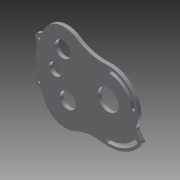
# Autodesk Inventor part: front plate
Saved by Autodesk Inventor 2012 (Build 160160000, 160)
## iProperties
Created: 2012-02-07
Part Number: front plate
Material: Default
Document SubType Name: Modeling
Designer: Antonella Wilby
Density: 1 g/cm^3
Author: Antonella Wilby
Autodesk Inventor part; units mm, degrees
ref_plane "YZ Plane" through (0, 0, 0) normal (1, 0, 0) x (0, 1, 0)
ref_plane "XZ Plane" through (0, 0, 0) normal (0, 1, 0) x (-1, 0, 0)
ref_plane "XY Plane" through (0, 0, 0) normal (0, 0, 1) x (1, 0, 0)
sketch "Sketch1" plane through (0, 0, 0) normal (0, 0, 1) x (1, 0, 0)
  line L0 (-198.2999, 0) -> (115.1427, 0) projected
  line L1 (0, -203.8942) -> (0, 193.807) projected
  circle A0 centre (0, 0) radius 53.975 construction
  circle A1 centre (0, 0) radius 19.05
  arc A2 (50.8401, -18.1268) -> (-4.087, 53.82) centre (0, 0) ccw
  line L2 (51.6197, -23.9016) -> (59.4633, -35.1034)
  arc A3 (50.8401, -18.1268) -> (51.6197, -23.9016) centre (56.8213, -20.2594) ccw
  line L3 (0, 0) -> (-57.7807, -26.9436) construction
  circle A4 centre (0, 0) radius 53.975 construction
  circle A5 centre (-95.7467, 0) radius 11.1125
  circle A6 centre (-73.1257, -37.5239) radius 14.2875
  circle A7 centre (-82.0671, 38.2685) radius 14.2875
  arc A8 (-56.7688, 67.6544) -> (-118.11, 48.895) centre (-79.7827, 33.238) ccw
  arc A9 (-118.11, -50.8) -> (-59.2151, -78.8871) centre (-77.6901, -41.8358) ccw
  arc A10 (-12.3378, -71.9752) -> (-59.2151, -78.8871) centre (-25.2121, -147.0797) ccw
  circle A11 centre (0, 0) radius 16.51 construction
  line L4 (0, 0) -> (-82.0671, 38.2685) construction
  circle A12 centre (-125.73, 34.29) radius 6.35 construction
  circle A13 centre (-125.73, -34.29) radius 6.35 construction
  line L5 (0, 0) -> (-34.422, 64.7383) construction
  line L6 (0, 0) -> (-56.7688, 67.6544) construction
  arc A14 (-127.2193, 41.2768) -> (-132.0785, 31.0144) centre (-125.73, 34.29) ccw
  arc A15 (-130.3268, 13.3001) -> (-130.3268, -13.3001) centre (-83.9357, 0) ccw
  arc A16 (-130.3268, 13.3001) -> (-132.0785, 31.0144) centre (-153.5223, 19.9501) ccw
  arc A17 (-132.0785, -31.0144) -> (-127.4503, -41.2235) centre (-125.73, -34.29) ccw
  arc A18 (-132.0785, -31.0144) -> (-130.3268, -13.3001) centre (-153.5223, -19.9501) ccw
  arc A19 (-118.11, -50.8) -> (-127.4503, -41.2235) centre (-130.5087, -53.5498) ccw
  arc A20 (-127.2193, 41.2768) -> (-118.11, 48.895) centre (-129.8669, 53.6978) ccw
  line L7 (-198.2999, 0) -> (115.1427, 0) projected
  line L8 (0, 193.807) -> (0, -203.8942) projected
  line L9 (-118.11, -50.8) -> (0, -50.8) construction
  arc A21 (-12.3378, -71.9752) -> (59.4295, -42.4357) centre (0, 0) ccw
  arc A22 (59.4295, -42.4357) -> (59.4633, -35.1034) centre (54.2617, -38.7456) ccw
  line L10 (0, 0) -> (41.8854, -59.8186) construction
  line L11 (-118.11, 48.895) -> (0, 48.895) construction
  arc A23 (-56.7688, 67.6544) -> (-4.087, 53.82) centre (-10.4031, 136.9926) ccw
  point P0 (61.9528, -38.6588)
  point P1 (-67.9722, -26.6913)
  dimension "d67" = 107.95
  dimension "d68" = 38.1
  dimension "d84" = 65
  dimension "d88" = 107.95
  dimension "d89" = 22.225
  dimension "d90" = 28.575
  dimension "d99" = 33.02
  dimension "d100" = 43.815
  dimension "d103" = 28.575
  dimension "d105" = 90.551
  dimension "d106" = 12.7
  dimension "d107" = 12.7
  dimension "d114" = 14.2875
  dimension "d115" = 14.2875
  dimension "d117" = 24.13
  dimension "d118" = 24.13
  dimension "d119" = 48.26
  dimension "d120" = 12.7
  dimension "d124" = 76.2
  dimension "d127" = 28
  dimension "d128" = 40
  dimension "d129" = 65
  dimension "d130" = 40.64
  dimension "d131" = 34.29
  dimension "d132" = 34.29
  dimension "d133" = 125.73
  dimension "d134" = 125.73
  dimension "d138" = 11.811
  dimension "d140" = 50.8
  dimension "d141" = 118.11
  dimension "d153" = 35
  dimension "d154" = 6.35
  dimension "d155" = 6.35
  dimension "d167" = 73.025
  dimension "d168" = 28.575
  dimension "d169" = 12.7
  dimension "d170" = 41.402
  dimension "d173" = 118.11
  dimension "d174" = 48.895
  constraints: 32 point on circle, 24 centre point, 17 tangent, 16 end point, 12 coincident, 3 point on line, 2 horizontal alignment, 2 perpendicular, 1 equal radius, 1 parallel
  measures "d67" diameter of A0
  measures "d68" diameter of A1
  measures "d84" angle of L3 L1
  measures "d88" diameter of A4
  measures "d89" diameter of A5
  measures "d90" diameter of A7
  measures "d99" diameter of A11
  measures "d100" distance of A6.centre A5.centre
  measures "d103" diameter of A6
  measures "d105" distance of L4.start L4.end
  measures "d106" diameter of A12
  measures "d107" diameter of A13
  measures "d114" diameter of A14
  measures "d115" diameter of A17
  measures "d117" radius of A16
  measures "d118" radius of A18
  measures "d119" radius of A15
  measures "d120" radius of A19
  measures "d124" radius of A10
  measures "d127" angle of L8 L5
  measures "d128" angle of L8 L6
  measures "d129" angle of L8 L4
  measures "d130" distance of A7.centre A5.centre
  measures "d131" distance from line of A12.centre L7
  measures "d132" distance from line of A13.centre L7
  measures "d133" distance from line of L8 A12.centre
  measures "d134" distance from line of L8 A13.centre
  measures "d138" distance of A5.centre A15.centre
  measures "d140" distance between parallel lines of L7 L9
  measures "d141" distance of L9.start L9.end
  measures "d153" angle of L2 L8
  measures "d154" radius of A22
  measures "d155" radius of A3
  measures "d167" radius of A21
  measures "d168" distance between parallel lines of L2 L10
  measures "d169" radius of A20
  measures "d170" radius of A8
  measures "d173" distance of L11.start L11.end
  measures "d174" distance between parallel lines of L11 L0
extrude "Base" add sketch "Sketch1" along normal mid plane 6.35 contours A15 A16 A14 A20 A8 A23 A2 L1 A1 L0 A5 | L0 A5 A1 L1 A21 A10 A9 A19 A17 A18 A15 | L1 A2 L0 A1 | A1 L0 A2 A3 L2 A22 A21 L1
sketch "Sketch2" plane through (0, 0, -3.175) normal (0, 0, -1) x (-1, 0, 0)
  arc A0 (127.4503, -41.2235) -> (132.0785, -31.0144) centre (125.73, -34.29) ccw projected
  arc A1 (132.0785, 31.0144) -> (127.2193, 41.2768) centre (125.73, 34.29) ccw projected
  constraints: 2 coincident
hole "Standoff holes to back plate" at (-125.73, 34.29, -3.175) at (-125.73, -34.29, -3.175) direction (0, 0, 1) diameter 5.1054 end through all counterbore diameter 9.779 counterbore depth 1.5875 clearance for "Flat Head Machine Screw (82)" size "#10" standard "Ansi Unified Screw Threads"
sketch "Sketch3" plane through (0, 0, 3.175) normal (0, 0, 1) x (1, 0, 0)
  arc A0 (-12.3378, -71.9752) -> (59.4295, -42.4357) centre (0, 0) ccw projected
  line L0 (51.6197, -23.9016) -> (59.4633, -35.1034) projected
  arc A1 (50.8401, -18.1268) -> (-4.087, 53.82) centre (0, 0) ccw projected
  line L1 (-173.5215, 0) -> (111.013, 0) projected
  line L2 (0, -114.8134) -> (0, 106.2156) projected
  arc A2 (0, -61.5061) -> (47.1164, -39.5354) centre (0, 0) ccw
  arc A3 (52.2921, -43.8783) -> (47.1164, -39.5354) centre (49.7043, -41.7068) ccw
  arc A4 (0, -61.5061) -> (0, -68.2625) centre (0, -64.8843) ccw
  arc A5 (0, -68.2625) -> (52.2921, -43.8783) centre (0, 0) ccw
  line L3 (49.7043, -41.7068) -> (0, 0) construction
  line L4 (0, -64.8843) -> (0, 0) construction
  point P0 (-10.4819, 52.9474)
  dimension "d159" = 4.7625
  dimension "d160" = 6.7564
  dimension "d161" = 15
  dimension "d162" = 50
  constraints: 8 point on circle, 4 centre point, 4 end point, 4 tangent
  measures "d159" radial gap between concentric circles of A5 A0
  measures "d160" radial gap between concentric circles of A2 A5
  measures "d161" angle of L0 L3
  measures "d162" angle of L3 L4
extrude "Tensioning Slot" cut sketch "Sketch3" against normal through all contours A2 A3 A5 L2 | L2 A4
sketch "Sketch4" plane through (0, 0, 3.175) normal (0, 0, 1) x (1, 0, 0)
  arc A0 (50.8401, -18.1268) -> (-4.087, 53.82) centre (0, 0) ccw projected
  arc A1 (-12.3378, -71.9752) -> (59.4295, -42.4357) centre (0, 0) ccw projected
  line L0 (-173.5215, 0) -> (111.013, 0) projected
  line L1 (0, -114.8134) -> (0, 106.2156) projected
  arc A2 (41.8111, 7.3724) -> (48.4649, 8.5457) centre (45.138, 7.959) ccw
  arc A3 (4.2892, 49.0252) -> (3.7003, 42.2945) centre (3.9947, 45.6599) ccw
  arc A4 (41.8111, 7.3724) -> (3.7003, 42.2945) centre (0, 0) ccw
  arc A5 (48.4649, 8.5457) -> (4.2892, 49.0252) centre (0, 0) ccw
  line L2 (0, 0) -> (3.9947, 45.6599) construction
  line L3 (0, 0) -> (45.138, 7.959) construction
  dimension "d181" = 4.7625
  dimension "d182" = 6.7564
  dimension "d183" = 75
  dimension "d187" = 10
  constraints: 8 point on circle, 4 centre point, 4 end point, 4 tangent
  measures "d181" radial gap between concentric circles of A0 A5
  measures "d182" radial gap between concentric circles of A5 A4
  measures "d183" angle of L2 L3
  measures "d187" angle of L3 L0
extrude "Tensioning Slot:2" cut sketch "Sketch4" against normal through all contours A4 A3 A5 A2
equation "\"d132\" = d131"
equation "\"d134\" = d133"
body "Solid1"
